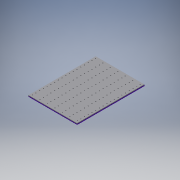
# Autodesk Inventor part: KrackenPlate2
Saved by Autodesk Inventor 2016 (Build 200138000, 138)
## iProperties
Created: 2015-09-06
Part Number: KrackenPlate2
Material: Generic
Document SubType Name: Modeling
Designer: Tim
Density: 1 g/cm^3
Appearance: Default
Author: Tim
Autodesk Inventor part; units mm, degrees
ref_plane "YZ Plane" through (0, 0, 0) normal (1, 0, 0) x (0, 1, 0)
ref_plane "XZ Plane" through (0, 0, 0) normal (0, 1, 0) x (-1, 0, 0)
ref_plane "XY Plane" through (0, 0, 0) normal (0, 0, 1) x (1, 0, 0)
sketch "Sketch1" plane through (0, 0, 0) normal (0, 0, 1) x (1, 0, 0)
  line L0 (104, -144) -> (-104, -144)
  line L1 (-104, -144) -> (-104, 144)
  line L2 (-104, 144) -> (104, 144)
  line L3 (104, 144) -> (104, -144)
  line L4 (104, -144) -> (-104, 144) construction
  line L5 (-104, -144) -> (104, 144) construction
  circle A0 centre (96, 134.4) radius 1.85
  circle A1 centre (64, 134.4) radius 1.85
  circle A2 centre (32, 134.4) radius 1.85
  circle A3 centre (0, 134.4) radius 1.85
  circle A4 centre (-32, 134.4) radius 1.85
  circle A5 centre (-64, 134.4) radius 1.85
  circle A6 centre (-96, 134.4) radius 1.85
  circle A7 centre (64, -134.4) radius 1.85
  circle A8 centre (32, -134.4) radius 1.85
  circle A9 centre (96, -134.4) radius 1.85
  circle A10 centre (0, -134.4) radius 1.85
  circle A11 centre (-32, -134.4) radius 1.85
  circle A12 centre (-96, -134.4) radius 1.85
  line L6 (104, 144) -> (-104, -144) construction
  line L7 (-104, 144) -> (104, -144) construction
  circle A13 centre (-64, -134.4) radius 1.85
  circle A14 centre (0, -8) radius 1.85 projected
  circle A15 centre (0, 8) radius 1.85 projected
  circle A16 centre (-96, 8) radius 1.85 projected
  circle A17 centre (-96, -8) radius 1.85 projected
  circle A18 centre (96, 8) radius 1.85 projected
  circle A19 centre (96, -8) radius 1.85 projected
  circle A20 centre (64, -8) radius 1.85 projected
  circle A21 centre (64, 8) radius 1.85 projected
  circle A22 centre (32, -8) radius 1.85 projected
  circle A23 centre (32, 8) radius 1.85 projected
  circle A24 centre (-32, -8) radius 1.85 projected
  circle A25 centre (-32, 8) radius 1.85 projected
  circle A26 centre (-64, -8) radius 1.85 projected
  circle A27 centre (-64, 8) radius 1.85 projected
  circle A28 centre (-96, 120) radius 1.85 projected
  circle A29 centre (-96, 104) radius 1.85 projected
  circle A30 centre (-96, 88) radius 1.85 projected
  circle A31 centre (-96, 56) radius 1.85 projected
  circle A32 centre (-96, 40) radius 1.85 projected
  circle A33 centre (-96, 24) radius 1.85 projected
  circle A34 centre (-64, 24) radius 1.85 projected
  circle A35 centre (-64, 56) radius 1.85 projected
  circle A36 centre (-64, 40) radius 1.85 projected
  circle A37 centre (-64, 88) radius 1.85 projected
  circle A38 centre (-64, 72) radius 1.85 projected
  circle A39 centre (-64, 120) radius 1.85 projected
  circle A40 centre (-64, 104) radius 1.85 projected
  circle A41 centre (-32, 120) radius 1.85 projected
  circle A42 centre (-32, 104) radius 1.85 projected
  circle A43 centre (-32, 88) radius 1.85 projected
  circle A44 centre (-32, 72) radius 1.85 projected
  circle A45 centre (0, 88) radius 1.85 projected
  circle A46 centre (0, 104) radius 1.85 projected
  circle A47 centre (0, 120) radius 1.85 projected
  circle A48 centre (32, 120) radius 1.85 projected
  circle A49 centre (32, 104) radius 1.85 projected
  circle A50 centre (64, 120) radius 1.85 projected
  circle A51 centre (64, 104) radius 1.85 projected
  circle A52 centre (64, 88) radius 1.85 projected
  circle A53 centre (32, 88) radius 1.85 projected
  circle A54 centre (32, 72) radius 1.85 projected
  circle A55 centre (64, 72) radius 1.85 projected
  circle A56 centre (0, 72) radius 1.85 projected
  circle A57 centre (-32, 56) radius 1.85 projected
  circle A58 centre (-32, 40) radius 1.85 projected
  circle A59 centre (0, 56) radius 1.85 projected
  circle A60 centre (0, 40) radius 1.85 projected
  circle A61 centre (32, 56) radius 1.85 projected
  circle A62 centre (32, 40) radius 1.85 projected
  circle A63 centre (64, 56) radius 1.85 projected
  circle A64 centre (64, 40) radius 1.85 projected
  circle A65 centre (64, 24) radius 1.85 projected
  circle A66 centre (32, 24) radius 1.85 projected
  circle A67 centre (0, 24) radius 1.85 projected
  circle A68 centre (-32, 24) radius 1.85 projected
  circle A69 centre (-96, 72) radius 1.85 projected
  circle A70 centre (64, -24) radius 1.85 projected
  circle A71 centre (64, -40) radius 1.85 projected
  circle A72 centre (32, -24) radius 1.85 projected
  circle A73 centre (32, -40) radius 1.85 projected
  circle A74 centre (32, -56) radius 1.85 projected
  circle A75 centre (64, -56) radius 1.85 projected
  circle A76 centre (64, -72) radius 1.85 projected
  circle A77 centre (32, -72) radius 1.85 projected
  circle A78 centre (0, -40) radius 1.85 projected
  circle A79 centre (0, -24) radius 1.85 projected
  circle A80 centre (0, -56) radius 1.85 projected
  circle A81 centre (0, -72) radius 1.85 projected
  circle A82 centre (-32, -24) radius 1.85 projected
  circle A83 centre (-64, -24) radius 1.85 projected
  circle A84 centre (-96, -24) radius 1.85 projected
  circle A85 centre (-96, -40) radius 1.85 projected
  circle A86 centre (-64, -40) radius 1.85 projected
  circle A87 centre (-32, -40) radius 1.85 projected
  circle A88 centre (-32, -56) radius 1.85 projected
  circle A89 centre (-64, -56) radius 1.85 projected
  circle A90 centre (-96, -56) radius 1.85 projected
  circle A91 centre (-96, -72) radius 1.85 projected
  circle A92 centre (-64, -72) radius 1.85 projected
  circle A93 centre (-32, -72) radius 1.85 projected
  circle A94 centre (-32, -88) radius 1.85 projected
  circle A95 centre (0, -88) radius 1.85 projected
  circle A96 centre (32, -88) radius 1.85 projected
  circle A97 centre (64, -88) radius 1.85 projected
  circle A98 centre (64, -104) radius 1.85 projected
  circle A99 centre (32, -104) radius 1.85 projected
  circle A100 centre (0, -104) radius 1.85 projected
  circle A101 centre (-32, -104) radius 1.85 projected
  circle A102 centre (-64, -104) radius 1.85 projected
  circle A103 centre (-64, -88) radius 1.85 projected
  circle A104 centre (-96, -88) radius 1.85 projected
  circle A105 centre (-96, -104) radius 1.85 projected
  circle A106 centre (-96, -120) radius 1.85 projected
  circle A107 centre (-64, -120) radius 1.85 projected
  circle A108 centre (-32, -120) radius 1.85 projected
  circle A109 centre (0, -120) radius 1.85 projected
  circle A110 centre (32, -120) radius 1.85 projected
  circle A111 centre (64, -120) radius 1.85 projected
  circle A112 centre (96, 56) radius 1.85 projected
  circle A113 centre (96, 40) radius 1.85 projected
  circle A114 centre (96, 24) radius 1.85 projected
  circle A115 centre (96, -24) radius 1.85 projected
  circle A116 centre (96, -40) radius 1.85 projected
  circle A117 centre (96, -72) radius 1.85 projected
  circle A118 centre (96, -88) radius 1.85 projected
  circle A119 centre (96, -104) radius 1.85 projected
  circle A120 centre (96, -120) radius 1.85 projected
  circle A121 centre (96, -56) radius 1.85 projected
  circle A122 centre (96, 120) radius 1.85 projected
  circle A123 centre (96, 104) radius 1.85 projected
  circle A124 centre (96, 88) radius 1.85 projected
  circle A125 centre (96, 72) radius 1.85 projected
  dimension "d0" = 208
  dimension "d1" = 288
  dimension "d17" = 32
  dimension "d18" = 32
  dimension "d19" = 32
  dimension "d20" = 32
  dimension "d21" = 32
  dimension "d22" = 32
  dimension "d23" = 8
  dimension "d25" = 9.6
  dimension "d26" = 9.6
  dimension "d27" = 8
  dimension "d29" = 9.6
  dimension "d30" = 8
  dimension "d31" = 14.4
  dimension "d32" = 16
  dimension "d33" = 14.4
  dimension "d34" = 14.4
  dimension "d35" = 16
  dimension "d36" = 14.4
  dimension "d37" = 16
  dimension "d38" = 16
  dimension "d39" = 9.6
  dimension "d40" = 8
  constraints: 16 end point, 2 parallel, 1 horizontal, 1 perpendicular
  measures "d0" distance of L2.start L2.end
  measures "d1" distance of L2.end L3.end
  measures "d17" distance of A13.centre A12.centre
  measures "d18" distance of A11.centre A13.centre
  measures "d19" distance of A11.centre A10.centre
  measures "d20" distance of A10.centre A8.centre
  measures "d21" distance of A7.centre A8.centre
  measures "d22" distance of A7.centre A9.centre
  measures "d23" distance from line of L1 A12.centre
  measures "d25" distance from line of L0 A12.centre
  measures "d26" distance from line of L0 A9.centre
  measures "d27" distance from line of L1 A6.centre
  measures "d29" distance from line of L2 A0.centre
  measures "d30" distance from line of L3 A0.centre
  measures "d31" distance of A106.centre A12.centre
  measures "d32" distance of A106.centre A105.centre
  measures "d33" distance of A28.centre A6.centre
  measures "d34" distance of A9.centre A120.centre
  measures "d35" distance of A119.centre A120.centre
  measures "d36" distance of A0.centre A122.centre
  measures "d37" distance of A122.centre A123.centre
  measures "d38" distance of A28.centre A29.centre
  measures "d39" distance from line of L2 A6.centre
  measures "d40" distance from line of L3 A9.centre
extrude "Extrusion8" add sketch "Sketch1" along normal blind 4
body "Solid8"
